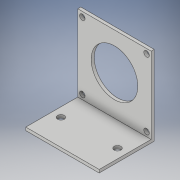
# Autodesk Inventor part: Motorhalterung
Saved by Autodesk Inventor 2019 (Build 230136000, 136)
## iProperties
Created: 2019-02-21
Part Number: Motorhalterung
Material: Generisch
Document SubType Name: Modeling
Designer: nico-
Density: 1 g/cm^3
Appearance: Vorgabe
Author: nico-
Autodesk Inventor part; units mm, degrees
ref_plane "YZ Plane" through (0, 0, 0) normal (1, 0, 0) x (0, 1, 0)
ref_plane "XZ Plane" through (0, 0, 0) normal (0, 1, 0) x (-1, 0, 0)
ref_plane "XY Plane" through (0, 0, 0) normal (0, 0, 1) x (1, 0, 0)
sketch "Skizze1" plane through (0, 0, 0) normal (1, 0, 0) x (0, 1, 0)
  line L0 (0, 0) -> (0, -45)
  line L1 (0, -45) -> (65, -45)
  line L2 (65, -45) -> (65, -42.5)
  line L3 (65, -42.5) -> (2.5, -42.5)
  line L4 (2.5, -42.5) -> (2.5, 0)
  line L5 (2.5, 0) -> (0, 0)
  dimension "d0" = 45
  dimension "d1" = 65
  dimension "d2" = 2.5
  dimension "d3" = 62.5
  constraints: 12 end point, 4 perpendicular, 2 vertical
  measures "d0" distance of L0.start L0.end
  measures "d1" distance of L0.end L1.end
  measures "d2" distance of L1.end L2.end
  measures "d3" distance of L2.end L3.end
extrude "Extrusion1" add sketch "Skizze1" along normal mid plane 60
sketch "Skizze2" plane through (-30, 2.5, 0) normal (0, 1, 0) x (1, 0, 0)
  circle A0 centre (7.5, 21.25) radius 2.75
  circle A1 centre (52.5, 22.5) radius 2.75
  point P0 (30, 0)
  dimension "d6" = 5.5
  dimension "d7" = 5.5
  constraints: 2 centre point
  measures "d6" diameter of A0
  measures "d7" diameter of A1
extrude "Extrusion2" cut sketch "Skizze2" against normal blind 3
sketch "Skizze3" plane through (-30, 2.5, -42.5) normal (0, 0, 1) x (1, 0, 0)
  circle A0 centre (30, 32.2) radius 19.075
  circle A1 centre (56.25, 58.75) radius 2.25
  line L0 (0, 62.5) -> (60, 62.5) projected
  circle A2 centre (3.75, 3.75) radius 2.25
  circle A3 centre (56.25, 3.75) radius 2.25
  circle A4 centre (3.75, 58.45) radius 2.25
  point P0 (30, -2.5)
  dimension "d10" = 38.15
  dimension "d11" = 4.5
  dimension "d12" = 3.75
  dimension "d13" = 4.5
  dimension "d14" = 4.5
  dimension "d15" = 4.5
  constraints: 5 centre point
  measures "d10" diameter of A0
  measures "d11" diameter of A1
  measures "d12" distance from line of A1.centre L0
  measures "d13" diameter of A2
  measures "d14" diameter of A3
  measures "d15" diameter of A4
extrude "Extrusion3" cut sketch "Skizze3" against normal blind 2.5
